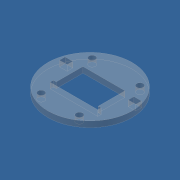
# Autodesk Inventor part: S1702_couverclereplat
Saved by Autodesk Inventor 2015 SP2 (Build 190223200, 223)
## iProperties
Created: 2017-10-31
Part Number: S1702_couverclereplat
Project: S1702_014_Circuit_Course
Material: Plastique PMMA
Description: Couvercle Interne
Document SubType Name: Modeling
Designer: Benoit.CURCHOD2
Authority: Ø44x3
Density: 1.188 g/cm^3
Appearance: Transparent - Clair
Mass: 3.97685 g
Surface Area: 30.9144 cm^2
Volume: 3.34752 cm^3
Material number: ---
Author: Benoit.CURCHOD2
Autodesk Inventor part; units mm, degrees
ref_plane "Plan YZ" through (0, 0, 0) normal (1, 0, 0) x (0, 1, 0)
ref_plane "Plan XZ" through (0, 0, 0) normal (0, 1, 0) x (-1, 0, 0)
ref_plane "Plan XY" through (0, 0, 0) normal (0, 0, 1) x (1, 0, 0)
sketch "Esquisse1" plane through (0, 0, 0) normal (0, 0, 1) x (1, 0, 0)
  circle A0 centre (0, 0) radius 22
  line L0 (12.5, -6.7) -> (12.5, -8.4)
  line L1 (12.5, -8.4) -> (-12.5, -8.4)
  line L2 (-12.5, -8.4) -> (-12.5, -6.7)
  line L3 (-11, -6.7) -> (-11, 7.3)
  line L4 (11, -6.7) -> (11, 7.3)
  line L5 (-12.5, -6.7) -> (-11, -6.7)
  line L6 (12.5, -6.7) -> (11, -6.7)
  line L7 (-11, 7.3) -> (11, 7.3)
  line L8 (-20, 7) -> (-16, 7)
  line L9 (-16, 7) -> (-16, 4)
  line L10 (-16, 4) -> (-20, 4)
  line L11 (-20, 4) -> (-20, 7)
  line L12 (20, 7) -> (16, 7)
  line L13 (16, 7) -> (16, 4)
  line L14 (16, 4) -> (20, 4)
  line L15 (20, 4) -> (20, 7)
  line L16 (-30.8, 0) -> (30.8, 0) construction
  line L17 (0, -30.8) -> (0, 30.8) construction
  circle A1 centre (-12.5, 13.6382) radius 1.7
  circle A2 centre (12.5, 13.6382) radius 1.7
  circle A3 centre (10, -15.5644) radius 1.7
  circle A4 centre (-10, -15.5644) radius 1.7
  circle A5 centre (0, 0) radius 18.5 construction
  dimension "d0" = 44
  dimension "d17" = 1.5
  dimension "d23" = 3
  dimension "d24" = 4
  dimension "d25" = 32
  dimension "d38" = 4
  dimension "d43" = 1.7
  dimension "d44" = 14
  dimension "d47" = 25
  dimension "d48" = 3.4
  dimension "d49" = 20
  dimension "d50" = 25
  dimension "d52" = 37
  dimension "d57" = 6.7
  constraints: 32 end point, 6 centre point, 4 parallel, 3 horizontal, 2 point on circle, 1 coincident, 1 equal radius, 1 perpendicular, 1 vertical, 9 other
  measures "d0" diameter of A0
  measures "d17" distance of L2.end L3.start
  measures "d23" distance of L8.end L9.end
  measures "d24" distance of L8.start L8.end
  measures "d25" distance between parallel lines of L13 L9
  measures "d38" distance between parallel lines of L16 L10
  measures "d43" distance of L1.end L2.end
  measures "d44" distance of L4.start L4.end
  measures "d47" distance of L0.end L1.end
  measures "d48" diameter of A1
  measures "d49" distance of A3.centre A4.centre
  measures "d50" distance of A2.centre A1.centre
  measures "d52" diameter of A5
  measures "d57" distance between parallel lines of L16 L5
extrude "Extrusion4" add sketch "Esquisse1" along normal blind 3
